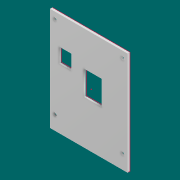
# Autodesk Inventor part: tappo ingeriore
Saved by Autodesk Inventor 2020 (Build 240168000, 168)
## iProperties
Created: 2025-01-02
Part Number: tappo ingeriore
Material: Plastica ABS
Document SubType Name: Modeling
Designer: Nicola Milia
Density: 1.06 g/cm^3
Appearance: Liscia - Bianco
Author: Nicola Milia
## iProperties of the stored document _Stampa 3D.ipt
Created: 2025-01-02
Part Number: _Stampa 3D
Material: Generico
Document SubType Name: Modeling
Designer: Nicola Milia
Density: 1 g/cm^3
Appearance: Default
Author: Nicola Milia
Autodesk Inventor part; units mm, degrees
ref_plane "YZ Plane" through (0, 0, 0) normal (1, 0, 0) x (0, 1, 0)
ref_plane "XZ Plane" through (0, 0, 0) normal (0, 1, 0) x (-1, 0, 0)
ref_plane "Piano di lavoro1" through (0, 0, 0) normal (0, 0, 1) x (1, 0, 0)
sketch "Schizzo1" plane through (0, 0, 0) normal (0, 0, 1) x (1, 0, 0)
  line L0 (16, 20.5) -> (-6, 20.5) projected
  line L1 (16, -9.5) -> (16, 20.5) projected
  line L2 (-6, -9.5) -> (16, -9.5) projected
  line L3 (-6, 20.5) -> (-6, -9.5) projected
  line L4 (-21, 10.5) -> (-21, 28.5) projected
  line L5 (-21, 28.5) -> (-36, 28.5) projected
  line L6 (-36, 10.5) -> (-21, 10.5) projected
  line L7 (-36, 28.5) -> (-36, 10.5) projected
  circle A0 centre (-41, 54.5) radius 2 projected
  circle A1 centre (41, 54.5) radius 2 projected
  circle A2 centre (41, -45.5) radius 2 projected
  circle A3 centre (-41, -45.5) radius 2 projected
  line L8 (47, -62.5) -> (-47, -62.5) projected
  line L9 (47, 62.5) -> (47, -62.5) projected
  line L10 (-47, 62.5) -> (47, 62.5) projected
  line L11 (-47, -62.5) -> (-47, 62.5) projected
  point P0 (0, 0)
extrude "Estrusione1" add sketch "Schizzo1" along normal blind 2
sketch "Schizzo2" plane through (0, 0, 0) normal (0, 0, -1) x (-1, 0, 0)
  line L0 (-47, -62.5) -> (-47, 62.5) projected
  line L1 (47, -62.5) -> (-47, -62.5) projected
  line L2 (47, 62.5) -> (47, -62.5) projected
  line L3 (-47, 62.5) -> (47, 62.5) projected
  circle A0 centre (41, 54.5) radius 2 projected
  circle A1 centre (-41, 54.5) radius 2 projected
  circle A2 centre (-41, -45.5) radius 2 projected
  circle A3 centre (41, -45.5) radius 2 projected
  line L4 (6, -9.5) -> (6, 20.5) projected
  line L5 (-16, -9.5) -> (6, -9.5) projected
  line L6 (-16, 20.5) -> (-16, -9.5) projected
  line L7 (6, 20.5) -> (-16, 20.5) projected
  line L8 (36, 10.5) -> (36, 28.5) projected
  line L9 (21, 10.5) -> (36, 10.5) projected
  line L10 (21, 28.5) -> (21, 10.5) projected
  line L11 (36, 28.5) -> (21, 28.5) projected
  point P0 (0, 0)
sketch "Schizzo3" plane through (0, 0, 0) normal (0, 0, -1) x (-1, 0, 0)
  line L0 (45, 60.5) -> (-45, 60.5) projected
  line L1 (-45, 60.5) -> (-45, -60.5) projected
  line L2 (45, -60.5) -> (45, 60.5) projected
  line L3 (-45, -60.5) -> (45, -60.5) projected
  point P0 (0, 0)
extrude "Estrusione2" cut sketch "Schizzo3" against normal blind 1
sketch "Schizzo4" plane through (-47, -62.5, 0) normal (0, -1, 0) x (1, 0, 0)
  line L0 (0, 0) -> (94, 0) projected
  line L1 (94, 0) -> (94, 2) projected
  line L2 (0, 2) -> (94, 2) projected
  line L3 (0, 0) -> (0, 2) projected
  line L4 (0, 0) -> (94, 0) projected
  line L5 (94, 0) -> (94, 2) projected
  line L6 (0, 2) -> (94, 2) projected
  line L7 (0, 0) -> (0, 2) projected
  point P0 (47, 0)
sketch "Schizzo5" plane through (0, 0, 2) normal (0, 0, 1) x (1, 0, 0)
  line L0 (47, -62.5) -> (47, 62.5) projected
  line L1 (47, 62.5) -> (-47, 62.5) projected
  line L2 (-47, 62.5) -> (-47, -62.5) projected
  line L3 (-47, -62.5) -> (47, -62.5) projected
  circle A0 centre (-41, 54.5) radius 2 projected
  circle A1 centre (41, 54.5) radius 2 projected
  circle A2 centre (41, -45.5) radius 2 projected
  circle A3 centre (-41, -45.5) radius 2 projected
  line L4 (-6, -9.5) -> (-6, 20.5) projected
  line L5 (-6, 20.5) -> (16, 20.5) projected
  line L6 (16, 20.5) -> (16, -9.5) projected
  line L7 (16, -9.5) -> (-6, -9.5) projected
  line L8 (-36, 10.5) -> (-36, 28.5) projected
  line L9 (-36, 28.5) -> (-21, 28.5) projected
  line L10 (-21, 28.5) -> (-21, 10.5) projected
  line L11 (-21, 10.5) -> (-36, 10.5) projected
  point P0 (0, 0)
extrude "Estrusione3" add sketch "Schizzo5" along normal blind 1
